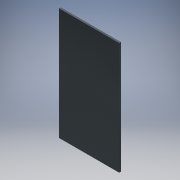
# Autodesk Inventor part: Plate Partition
Saved by Autodesk Inventor 2016 (Build 200138000, 138)
## iProperties
Created: 2018-11-10
Part Number: Plate Partition
Material: Steel ASTM A36
Document SubType Name: Modeling
Designer: asus
Density: 7.85 g/cm^3
Appearance: Plate - Blue
Mass: 14462.8 g
Surface Area: 4053.2 cm^2
Volume: 1842.39 cm^3
Author: asus
Autodesk Inventor part; units mm, degrees
ref_plane "YZ Plane" through (0, 0, 0) normal (1, 0, 0) x (0, 1, 0)
ref_plane "XZ Plane" through (0, 0, 0) normal (0, 1, 0) x (-1, 0, 0)
ref_plane "XY Plane" through (0, 0, 0) normal (0, 0, 1) x (1, 0, 0)
sketch "Sketch2" plane through (0, 0, 0) normal (0, 0, 1) x (1, 0, 0)
  line L0 (-161.0298, 4.75) -> (161.0298, 4.75)
  line L1 (161.0298, -4.75) -> (-161.0298, -4.75)
  arc A0 (-161.0298, 4.75) -> (-161.0298, -4.75) centre (0, 0) ccw
  arc A1 (161.0298, -4.75) -> (161.0298, 4.75) centre (0, 0) ccw
  point P0 (0, 4.75)
  point P1 (0, -4.75)
  point P2 (-161.0999, 0)
  dimension "d4" = 9.5
  dimension "d5" = 322.0597
  dimension "d7" = 322.0597
  constraints: 5 point on circle, 4 end point, 2 centre point, 2 coincident, 2 midpoint, 2 point on line, 2 vertical alignment, 1 horizontal alignment
  measures "d4" distance between parallel lines of L1 L0
  measures "d5" distance of L1.start L1.end
  measures "d7" distance of L0.start L0.end
extrude "Extrusion1" add sketch "Sketch2" along normal blind 301 and the other way blind 301
body "Solid1"
